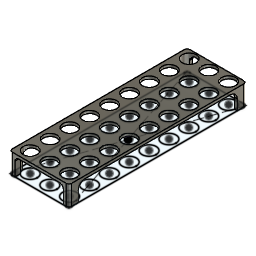
12Ga Holder v5 (Autodesk Fusion 360 design; units mm, degrees)
Autodesk Fusion 360 part; units mm, degrees
sketch "Sketch1" plane through (0, 0, 0) normal (0, 0, 1) x (1, 0, 0)
  line L0 (39, 128.5) -> (-39, 128.5)
  line L1 (-43, 124.5) -> (-43, -124.5)
  line L2 (-39, -128.5) -> (39, -128.5)
  line L3 (43, -124.5) -> (43, 124.5)
  line L4 (43, 128.5) -> (-43, -128.5) construction
  line L5 (-43, 128.5) -> (43, -128.5) construction
  arc A0 (-39, 128.5) -> (-43, 124.5) centre (-39, 124.5) ccw
  arc A1 (43, 124.5) -> (39, 128.5) centre (39, 124.5) ccw
  arc A2 (-43, -124.5) -> (-39, -128.5) centre (-39, -124.5) ccw
  arc A3 (39, -128.5) -> (43, -124.5) centre (39, -124.5) ccw
  circle A4 centre (-28, -113.5) radius 10.15
  circle A5 centre (0.5, -113.5) radius 10.15
  circle A6 centre (29, -113.5) radius 10.15
  circle A7 centre (-28, -84.75) radius 10.15
  circle A8 centre (0.5, -84.75) radius 10.15
  circle A9 centre (29, -84.75) radius 10.15
  circle A10 centre (-28, -56) radius 10.15
  circle A11 centre (0.5, -56) radius 10.15
  circle A12 centre (29, -56) radius 10.15
  circle A13 centre (-28, -27.25) radius 10.15
  circle A14 centre (0.5, -27.25) radius 10.15
  circle A15 centre (29, -27.25) radius 10.15
  circle A16 centre (-28, 1.5) radius 10.15
  circle A17 centre (0.5, 1.5) radius 10.15
  circle A18 centre (29, 1.5) radius 10.15
  circle A19 centre (-28, 30.25) radius 10.15
  circle A20 centre (0.5, 30.25) radius 10.15
  circle A21 centre (29, 30.25) radius 10.15
  circle A22 centre (-28, 59) radius 10.15
  circle A23 centre (0.5, 59) radius 10.15
  circle A24 centre (29, 59) radius 10.15
  circle A25 centre (-28, 87.75) radius 10.15
  circle A26 centre (0.5, 87.75) radius 10.15
  circle A27 centre (29, 87.75) radius 10.15
  circle A28 centre (-28, 116.5) radius 10.15
  circle A29 centre (0.5, 116.5) radius 10.15
  circle A30 centre (29, 116.5) radius 10.15
  dimension "d1" = 86
  dimension "d2" = 257
  dimension "d3" = 4
  dimension "d4" = 4
  dimension "d5" = 4
  dimension "d6" = 4
  dimension "d7" = 20.3
  dimension "d8" = 15
  dimension "d9" = 15
  dimension "d12" = 57
  dimension "d13" = 230
  constraint horizontal L0
  constraint perpendicular L0 L1
  constraint parallel L0 L2
  constraint parallel L1 L3
  constraint coincident L4 origin
  constraint coincident L5 origin
  constraint coincident L5.start L0
  constraint coincident L5.start L1
  constraint tangent L0 A0
  constraint tangent L1 A0
  constraint coincident L4.start L0
  constraint coincident L4.start L3
  constraint tangent L0 A1
  constraint tangent L3 A1
  constraint coincident L4.end L1
  constraint coincident L4.end L2
  constraint tangent L1 A2
  constraint tangent L2 A2
  constraint coincident L5.end L2
  constraint coincident L5.end L3
  constraint tangent L2 A3
  constraint tangent L3 A3
  measures "d1" distance of L4.end L5.end
  measures "d2" distance of L5.start L4.end
  measures "d3" radius of A0
  measures "d4" radius of A1
  measures "d5" radius of A2
  measures "d6" radius of A3
  measures "d7" diameter of A4
  measures "d8" distance of L1 A4.centre
  measures "d9" distance of L2 A4.centre
extrude "Extrude1" add sketch "Sketch1" along normal blind 29
sketch "Sketch2" plane through (43, 0, 0) normal (1, 0, 0) x (0, 1, 0)
  line L0 (-124.5, 0) -> (124.5, 0)
  line L1 (124.5, 0) -> (124.5, 29)
  line L2 (124.5, 29) -> (-124.5, 29)
  line L3 (-124.5, 29) -> (-124.5, 0)
  line L4 (-105, 25) -> (105, 25)
  line L5 (115, 15) -> (115, 0)
  line L6 (115, 0) -> (-115, 0)
  line L7 (-115, 0) -> (-115, 15)
  arc A0 (-105, 25) -> (-115, 15) centre (-105, 15) ccw
  arc A1 (115, 15) -> (105, 25) centre (105, 15) ccw
  dimension "d16" = 10
  dimension "d17" = 10
  dimension "d23" = 4
  constraint horizontal L4
  constraint vertical L5
  constraint horizontal L6
  constraint vertical L7
  constraint coincident L0 L5.end
  constraint tangent L4 A0
  constraint tangent L7 A0
  constraint tangent L4 A1
  constraint tangent L5 A1
  measures "d16" radius of A0
  measures "d17" radius of A1
  measures "d23" distance of L2 L4
extrude "Extrude2" cut sketch "Sketch2" against normal blind 100 contours L0 L4 L5 L6 L7 A0 A1
sketch "Sketch3" plane through (0, -128.5, 0) normal (0, -1, 0) x (1, 0, 0)
  line L0 (-39, 0) -> (39, 0)
  line L1 (39, 0) -> (39, 29)
  line L2 (39, 29) -> (-39, 29)
  line L3 (-39, 29) -> (-39, 0)
  line L4 (-29.9335, 25) -> (29.7744, 25)
  line L5 (34.7744, 20) -> (34.7744, 0)
  line L6 (34.7744, 0) -> (-34.9335, 0)
  line L7 (-34.9335, 0) -> (-34.9335, 20)
  arc A0 (-29.9335, 25) -> (-34.9335, 20) centre (-29.9335, 20) ccw
  arc A1 (34.7744, 20) -> (29.7744, 25) centre (29.7744, 20) ccw
  dimension "d20" = 5
  dimension "d24" = 4
  constraint horizontal L4
  constraint vertical L5
  constraint horizontal L6
  constraint vertical L7
  constraint coincident L0 L5.end
  constraint tangent L4 A0
  constraint tangent L7 A0
  constraint tangent L4 A1
  constraint tangent L5 A1
  constraint equal A0 A1
  measures "d20" radius of A0
  measures "d24" distance of L2 L4
extrude "Extrude3" cut sketch "Sketch3" against normal blind 270 contours L0 L4 L5 L6 L7 A0 A1
equation "d14 = ( 58 / 2 ) * 1 mm"
named bodies: "12Ga Shell Holder"
